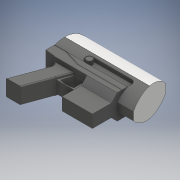
# Autodesk Inventor part: Sci-Fi Raycasting weapon
Saved by Autodesk Inventor 2017 (Build 210142000, 142)
## iProperties
Created: 2019-09-03
Part Number: Sci-Fi Raycasting weapon
Material: Generic
Document SubType Name: Modeling
Designer: Victor
Density: 1 g/cm^3
Appearance: Default
Author: Victor
Autodesk Inventor part; units mm, degrees
ref_plane "YZ Plane" through (0, 0, 0) normal (1, 0, 0) x (0, 1, 0)
ref_plane "XZ Plane" through (0, 0, 0) normal (0, 1, 0) x (-1, 0, 0)
ref_plane "XY Plane" through (0, 0, 0) normal (0, 0, 1) x (1, 0, 0)
sketch "Sketch1" plane through (0, 0, 0) normal (0, 0, 1) x (1, 0, 0)
  line L0 (0, 0) -> (-22, 0)
  line L1 (-22, 0) -> (-22, -5)
  line L2 (-22, -5) -> (0, -5)
  line L3 (0, -5) -> (0, 0)
  dimension "d0" = 22
  dimension "d1" = 5
  constraints: 8 end point, 3 perpendicular, 1 horizontal
  measures "d0" distance of L0.start L0.end
  measures "d1" distance of L0.end L1.end
extrude "Extrusion1" add sketch "Sketch1" along normal blind 7
sketch "Sketch2" plane through (0, -5, 0) normal (1, 0, 0) x (0, 0, -1)
  line L0 (0, 0) -> (0, 5) projected
  line L1 (-7, 5) -> (-7, 0) projected
  arc A0 (-4.5, 5) -> (-7, 0) centre (-0.7599, 0.0049) ccw
  arc A1 (0, 0) -> (-2.5, 5) centre (-6.2316, 0.0092) ccw
  line L2 (0, 5) -> (-7, 5) projected
  line L3 (-4.5, 5) -> (-7, 5)
  line L4 (-7, 5) -> (-7, 0)
  line L5 (-2.5, 5) -> (0, 5)
  line L6 (0, 5) -> (0, 0)
  dimension "d16" = 2.5
  dimension "d17" = 4.5
  dimension "d18" = 5
  dimension "d19" = 5
  dimension "d20" = 6.2316
  dimension "d21" = 6.2401
  constraints: 8 end point, 4 point on circle, 2 centre point
  measures "d16" distance from line of L0 L5.start
  measures "d17" distance from line of L0 L3.start
  measures "d18" vertical distance of L0.start L3.start
  measures "d19" vertical distance of L0.start L5.start
  measures "d20" radius of A1
  measures "d21" radius of A0
extrude "Extrusion3" cut sketch "Sketch2" against normal blind 40
sketch "Sketch4" plane through (-22, -5, 0) normal (0, -1, 0) x (1, 0, 0)
  line L0 (0, 0) -> (0, 7) projected
  line L1 (0, 7) -> (22, 7)
  line L2 (22, 7) -> (22, 0)
  line L3 (22, 0) -> (0, 0)
  line L4 (0, 0) -> (0, 7)
  constraints: 8 end point, 2 parallel, 1 horizontal, 1 perpendicular
extrude "Extrusion5" add sketch "Sketch4" along normal blind 5
sketch "Sketch5" plane through (0, -10, 7) normal (1, 0, 0) x (0, 0, -1)
  line L0 (0, 5) -> (0, 0) projected
  line L1 (7, 0) -> (0, 0) projected
  arc A0 (0, 4.9863) -> (2.5, 0) centre (6.2227, 4.9863) ccw
  line L2 (7, 5) -> (7, 0) projected
  arc A1 (4.5, 0) -> (7, 5) centre (-0.2236, 5.4868) ccw
  line L3 (0, 0) -> (7, 0) projected
  line L4 (2.5, 0) -> (0, 0)
  line L5 (0, 0) -> (0, 4.9863)
  line L6 (4.5, 0) -> (7, 0)
  line L7 (7, 0) -> (7, 5)
  point P0 (7, 10)
  dimension "d29" = 2.5
  dimension "d30" = 4.5
  dimension "d31" = 0
  dimension "d32" = 0
  dimension "d35" = 5.0137
  constraints: 8 end point, 4 point on circle, 2 centre point, 1 point on line
  measures "d29" distance from line of L0 L4.start
  measures "d30" distance from line of L6.start L0
  measures "d31" distance from line of L1 L6.start
  measures "d32" distance from line of L1 L4.start
  measures "d35" vertical distance of point (7, 10) A0.centre
extrude "Extrusion6" cut sketch "Sketch5" against normal blind 25
sketch "Sketch6" plane through (0, 0, 0) normal (0, 0, 1) x (1, 0, 0)
  line L0 (0, 0) -> (-2, 0)
  line L1 (0, 0) -> (0, -10)
  line L2 (0, -10) -> (-2, 0)
  dimension "d41" = 2
  dimension "d42" = 10
  constraints: 6 end point, 1 horizontal, 1 vertical
  measures "d41" distance of L0.start L0.end
  measures "d42" distance of L0.start L1.end
extrude "Extrusion7" cut sketch "Sketch6" along normal mid plane 40
ref_plane "Work Plane1" through (0, -11.2364, 0.7773) normal (0, -1, 0) x (1, 0, 0)
ref_plane "Work Plane2" through (-22, 0, 3.5) normal (-1, 0, 0) x (0, 0, 1)
sketch "Sketch7" plane through (-22, 0, 3.5) normal (-1, 0, 0) x (0, 0, 1)
  line L0 (1, -10) -> (-1, -10) projected
  line L1 (0, -7.5) -> (3.0581, -7.5)
  line L2 (3.0581, -7.5) -> (3.0581, -19.5)
  line L3 (3.0581, -19.5) -> (0, -19.5)
  line L4 (0, -19.5) -> (0, -7.5)
  line L5 (0, -7.5) -> (-3.0561, -7.5)
  line L6 (-3.0561, -7.5) -> (-3.0561, -19.5)
  line L7 (-3.0561, -19.5) -> (0, -19.5)
  line L8 (0, -19.5) -> (0, -7.5)
  point P0 (-3.5, 0)
  dimension "d45" = 2.5
  dimension "d46" = 3.5
  dimension "d47" = 12
  dimension "d48" = 12
  dimension "d122" = 3.0561
  dimension "d123" = 3.0581
  constraints: 16 end point, 4 parallel, 2 horizontal, 2 perpendicular
  measures "d45" distance from line of L0 L1.start
  measures "d46" horizontal distance of L1.start point (-3.5, 0)
  measures "d47" distance of L1.end L2.end
  measures "d48" distance of L6.end L5.end
  measures "d122" distance of L1.start L5.end
  measures "d123" distance of L1.start L1.end
extrude "Extrusion8" add sketch "Sketch7" against normal blind 18
sketch "Sketch8" plane through (-22, -19.5, 6.5581) normal (0, 0, 1) x (1, 0, 0)
  line L0 (0, 0) -> (18, 0) projected
  line L1 (0, 0) -> (7, 0) construction
  line L2 (0, 0) -> (0, 12) projected
  line L3 (0, 12) -> (0, 0) projected
  line L4 (0, 7.8783) -> (0, 0)
  line L5 (0, 0) -> (2.4483, 6.7267)
  line L6 (0, 7.8783) -> (0, 0)
  line L7 (2.4483, 6.7267) -> (2.9614, 8.1363)
  arc A0 (2.9614, 8.1363) -> (1.8029, 9.6293) centre (1.9122, 8.5181) ccw
  line L8 (1.8029, 9.6293) -> (0, 9.8637)
  line L9 (0, 9.8637) -> (0, 0)
  point P0 (22, 19.5)
  point P1 (0, 11.9999)
  point P2 (0, 11.9999)
  dimension "d60" = 70
  dimension "d73" = 1.5
  constraints: 14 end point, 2 collinear, 2 point on circle, 2 point on line, 1 centre point, 1 horizontal, 1 tangent
  measures "d60" angle of L0 L5
  measures "d73" distance of L5.end L7.end
extrude "Extrusion9" cut sketch "Sketch8" against normal blind 18
sketch "Sketch10" plane through (-22, -7.5001, 6.5581) normal (0, 0, 1) x (1, 0, 0)
  line L0 (6, -5.6504) -> (10.5112, -5.6504)
  line L1 (18, -9.9999) -> (18, -11.9999)
  line L2 (3.2721, -11.9999) -> (18, -11.9999)
  line L3 (10.5112, -5.6504) -> (10.5112, -8.6499)
  line L4 (10.5112, -8.6499) -> (18, -8.6499)
  line L5 (18, 0.0001) -> (18, -11.9999) projected
  line L6 (18, -8.6499) -> (18, -9.9999)
  line L7 (6, -5.6504) -> (3.689, -11.9999)
  line L8 (0, -11.9999) -> (18, -11.9999) projected
  line L9 (6, -5.6504) -> (12.757, -5.6504) construction
  line L10 (3.689, -11.9999) -> (18, -11.9999)
  point P0 (22, 7.5001)
  point P1 (18, 0)
  dimension "d79" = 12
  dimension "d80" = 110
  constraints: 18 end point, 3 horizontal, 2 perpendicular, 2 point on line, 1 collinear, 1 equal length, 1 vertical
  measures "d79" distance from line of L5 L0.start
  measures "d80" angle of L7 L9
extrude "Extrusion10" cut sketch "Sketch10" against normal blind 18
sketch "Sketch12" plane through (-22, -19.5, 0.4439) normal (0, -1, 0) x (1, 0, 0)
  line L0 (0, 5) -> (4, 5)
  line L1 (4, 0) -> (4, 6.1142) projected
  line L2 (0, 0) -> (0, 6.1142) projected
  line L3 (0, 1) -> (4, 1)
  line L4 (4, 5) -> (10.5112, 5)
  line L5 (10.5112, 6.1142) -> (10.5112, 0) projected
  line L6 (4, 1) -> (10.5112, 1)
  line L7 (0, 5) -> (0, 6.1142)
  line L8 (6.5112, 6.1142) -> (10.5112, 6.1142) projected
  line L9 (0, 6.1142) -> (10.5112, 6.1142)
  line L10 (10.5112, 6.1142) -> (10.5112, 5)
  line L11 (10.5112, 1) -> (10.5112, 0)
  line L12 (0, 0) -> (2.9614, 0) projected
  line L13 (10.5112, 0) -> (0, 0)
  line L14 (0, 0) -> (0, 1)
  point P0 (22, -0.4439)
  point P1 (3.4881, 0)
  constraints: 20 end point, 7 point on line, 5 perpendicular, 1 horizontal, 1 parallel, 1 vertical
extrude "Extrusion12" cut sketch "Sketch12" against normal blind 9.5 contours L2 L9 L1 L0 | L1 L9 L8 L5 L4 | L3 L1 L13 L12 L2 | L6 L5 L13 L1
sketch "Sketch15" plane through (-16, -13.1505, 1.4439) normal (0, -1, 0) x (1, 0, 0)
  line L0 (4.5112, 0) -> (4.5112, 0.5)
  line L1 (4.5112, 4) -> (4.5112, 0) projected
  line L2 (4.5112, 4) -> (4.5112, 3.5)
  line L3 (4.5112, 4) -> (4.5112, 3.5)
  line L4 (4.5112, 4) -> (1.1812, 4)
  line L5 (4.5112, 4) -> (0, 4) projected
  line L6 (1.1812, 4) -> (1.1812, 3.5)
  line L7 (1.1812, 3.5) -> (4.5112, 3.5)
  line L8 (4.5112, 0.5) -> (1.1812, 0.5)
  line L9 (1.1812, 0.5) -> (1.1812, 0)
  line L10 (0, 0) -> (4.5112, 0) projected
  line L11 (4.5112, 0) -> (1.1812, 0)
  point P0 (16, -1.4439)
  dimension "d88" = 3.33
  dimension "d89" = 0.5
  constraints: 18 end point, 4 perpendicular, 2 collinear, 2 point on line, 1 horizontal
  measures "d88" distance of L1.start L4.end
  measures "d89" distance of L4.end L6.end
extrude "Extrusion14" cut sketch "Sketch15" against normal blind 3.15
ref_plane "Work Plane4" through (-18.2929, -19.45, 5.4439) normal (0.9396926, -0.3420201, 0) x (-0.3420201, -0.9396926, 0)
sketch "Sketch19" plane through (-18.2929, -19.45, 5.4439) normal (0.9396926, -0.3420201, 0) x (-0.3420201, -0.9396926, 0)
  line L0 (-10.0565, 0) -> (-10.0565, 0.5)
  line L1 (-10.0565, 0.5) -> (-6.7065, 0.5)
  line L2 (-6.7065, 0) -> (-10.0565, 0)
  line L3 (-8.448, 0) -> (-7.3435, 0) projected
  line L4 (-6.7065, 0) -> (-6.7065, 0.5)
  line L5 (-10.0565, 4) -> (-10.0565, 3.5)
  line L6 (-10.0565, 3.5) -> (-6.7065, 3.5)
  line L7 (-6.7065, 3.5) -> (-6.7065, 4)
  line L8 (-6.7065, 4) -> (-10.0565, 4)
  point P0 (-24.5336, 5.4439)
  dimension "d90" = 0.5
  dimension "d91" = 90
  dimension "d92" = 3.35
  dimension "d93" = 3.35
  dimension "d94" = 0.5
  constraints: 16 end point, 3 perpendicular, 2 vertical, 1 collinear
  measures "d90" distance of L0.start L0.end
  measures "d91" angle of L0 L1
  measures "d92" distance of L0.end L1.end
  measures "d93" distance of L2.start L0.start
  measures "d94" distance of L5.start L5.end
extrude "Extrusion15" cut sketch "Sketch19" along normal blind 3.15
sketch "Sketch20" plane through (-14.8188, -10.0005, 4.9439) normal (0, 0, 1) x (1, 0, 0)
  arc A0 (-0.5426, -2.7207) -> (2.8171, -2.7457) centre (1.1783, 2.7917) ccw
  line L0 (2.8171, -2.7457) -> (2.8171, -0.1104)
  line L1 (2.8171, -0.1104) -> (0.2723, -0.1104)
  line L2 (0.2723, -0.1104) -> (-0.5426, -2.7207)
  point P0 (14.8188, 10.0005)
  constraints: 6 end point, 2 point on circle, 1 centre point, 1 perpendicular, 1 vertical
extrude "Extrusion16" cut sketch "Sketch20" against normal blind 3.15
ref_plane "Work Plane5" through (0, -5.0137, 7) normal (0, 0, 1) x (1, 0, 0)
sketch "Sketch22" plane through (0, -5.0137, 7) normal (0, 0, 1) x (1, 0, 0)
  arc A0 (-14.4382, -0.7422) -> (-14.4382, -2.4864) centre (-14.4382, -1.6143) ccw
  line L0 (-22, -2.4864) -> (-4, -2.4864) projected
  line L1 (-14.4382, -2.4864) -> (-4.6217, -2.4864)
  arc A1 (-4.6217, -2.4864) -> (-4.6217, -0.7422) centre (-4.6217, -1.6143) ccw
  line L2 (-4.6217, -0.7422) -> (-14.4382, -0.7422)
  point P0 (0, 5.0137)
  constraints: 4 end point, 4 point on circle, 4 tangent, 2 centre point, 2 point on line
extrude "Extrusion17" cut sketch "Sketch22" against normal blind 1
sketch "Sketch23" plane through (0, -5.0137, 6) normal (0, 0, 1) x (1, 0, 0)
  line L0 (-4.6217, -2.4864) -> (-14.4382, -2.4864) projected
  line L1 (-14.4382, -0.7422) -> (-4.6217, -0.7422) projected
  circle A0 centre (-14.2769, -1.6143) radius 0.7343
  point P0 (0, 5.0137)
  dimension "d102" = 0.8721
  dimension "d103" = 1.7442
  constraints: 1 centre point, 1 coincident
  measures "d102" distance from line of L0 point (-14.277, -1.614)
  measures "d103" distance between parallel lines of L0 L1
extrude "Extrusion18" add sketch "Sketch23" along normal blind 1
sketch "Sketch24" plane through (-22, -9.6363, 6.5581) normal (0, 0, 1) x (1, 0, 0)
  line L0 (0, 0) -> (0, 2.1363) projected
  line L1 (0, 2.1362) -> (2.9168, 2.1362)
  line L2 (18, 2.1362) -> (0, 2.1362) projected
  line L3 (2.9168, 2.1362) -> (7.0602, 0.8523)
  line L4 (7.0602, 0.8523) -> (18, 0.8522)
  line L5 (18, 2.1363) -> (18, -6.5137) projected
  line L6 (18, 0.7522) -> (7.045, 0.7523)
  line L7 (7.045, 0.7523) -> (2.9017, 2.0362)
  line L8 (2.9017, 2.0362) -> (0.1, 2.0362)
  line L9 (0.1, 2.0362) -> (0.1, 0)
  line L10 (0.1, 2.0362) -> (0, 2.0362)
  line L11 (0, 2.0362) -> (0, 2.1362)
  line L12 (18, 0.8522) -> (18, 0.7522)
  point P0 (22, 9.6363)
  point P1 (18, 2.1362)
  dimension "d106" = 0.1
  constraints: 20 end point, 4 point on line, 2 parallel, 1 collinear, 3 other
  measures "d106" distance between parallel lines of L4 L6
extrude "Extrusion19" cut sketch "Sketch24" against normal blind 0.8 contours L0 L1 L3 L4 L5 L6 L7 L8 L10
sketch "Sketch25" plane through (-4, 0, 3.5) normal (1, 0, 0) x (0, 0, -1)
  line L0 (-2.2581, -8.8841) -> (-3.0581, -8.8841) projected
  line L1 (-1.5581, -16.15) -> (-3.0581, -16.15)
  line L2 (-3.0581, -10) -> (-1.9439, -10) projected
  line L3 (-3.0581, -10) -> (-1.5581, -11.4241)
  line L4 (3.0561, -16.15) -> (1.5561, -16.15)
  line L5 (-3.0581, -16.15) -> (3.0561, -16.15) projected
  line L6 (3.0561, -16.15) -> (3.0561, -10) projected
  line L7 (3.0561, -16.15) -> (3.0561, -10)
  line L8 (1.5561, -16.15) -> (1.5561, -11.4241)
  line L9 (3.0561, -10) -> (2.0561, -10) projected
  line L10 (1.5561, -11.4241) -> (3.0561, -10)
  line L11 (-3.0581, -16.15) -> (-3.0581, -10)
  line L12 (-1.5581, -16.15) -> (-1.5581, -11.4241)
  point P0 (3.5, 0)
  point P1 (-2.3742, -8.8841)
  dimension "d111" = 1.5
  dimension "d112" = 4.7259
  dimension "d113" = 1.4241
  dimension "d114" = 1.5
  dimension "d115" = 4.7259
  dimension "d116" = 1.4241
  constraints: 16 end point, 1 collinear, 1 horizontal, 1 parallel, 1 perpendicular, 1 vertical
  measures "d111" distance of L1.start L1.end
  measures "d112" distance of L3.end L1.start
  measures "d113" vertical distance of L2.start L3.end
  measures "d114" distance of L4.start L4.end
  measures "d115" distance of L4.end L8.end
  measures "d116" vertical distance of L8.end L6.end
extrude "Extrusion21" cut sketch "Sketch25" against normal blind 7.5
sketch "Sketch26" plane through (-4, -7.5001, 0.4439) normal (0, 0, -1) x (-1, 0, 0)
  line L0 (18, 0) -> (15.0832, 0) projected
  line L1 (18, 0) -> (15.0832, 0)
  line L2 (10.9398, -1.2839) -> (0, -1.284) projected
  line L3 (15.0832, 0) -> (10.9398, -1.2839)
  line L4 (10.9398, -1.2839) -> (0, -1.284)
  line L5 (0, -1.384) -> (0, -2.4999) projected
  line L6 (0, -1.284) -> (0, -1.384)
  line L7 (0, -1.384) -> (10.955, -1.3839)
  line L8 (15.0983, -0.1) -> (18, -0.1) projected
  line L9 (10.955, -1.3839) -> (15.0983, -0.1)
  line L10 (15.0983, -0.1) -> (18, -0.1)
  line L11 (18, -0.1) -> (18, 0) projected
  line L12 (18, -0.1) -> (18, 0)
  point P0 (-4, 7.5001)
  constraints: 16 end point, 3 collinear, 1 horizontal, 1 parallel, 1 perpendicular
extrude "Extrusion22" cut sketch "Sketch26" against normal blind 0.8
fillet "Fillet1" radius 0.25 14 edges at (-14.8544, -10, 5.4439) (-15.4282, -11.5736, 5.4439) (-14.8553, -9.9996, 5.4439) (-14.8542, -9.9996, 5.4439) (-17.1555, -16.3252, 5.4439) (-19.044, -10.5856, 5.4439) (-20.5193, -15.4319, 5.4439) (-19.044, -10.5856, 1.4439) (-20.5193, -15.4319, 1.4439) (-14.8544, -10, 1.4439) (-14.8542, -9.9996, 1.4439) (-15.4282, -11.5736, 1.4439) (-14.8553, -9.9996, 1.4439) (-17.1555, -16.3252, 1.4439)
equation "\"d19\" = d18"
equation "\"d93\" = d92"
equation "\"d102\" = 0.5 * d103"
equation "\"d114\" = d111"
equation "\"d115\" = d112"
body "Solid1"
